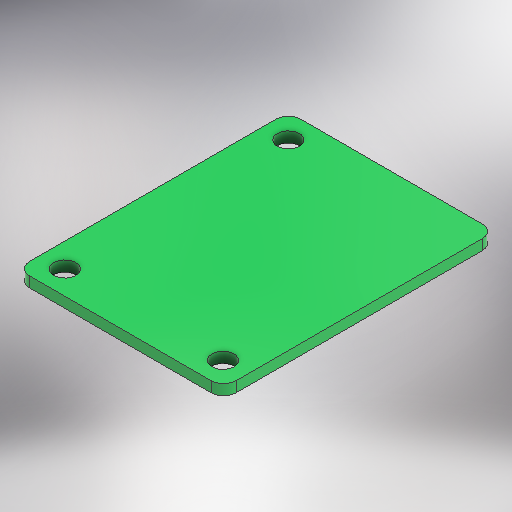
# Autodesk Inventor part: microphone_mcu
Saved by Autodesk Inventor 2026 (Build 300175050, 175E)
## iProperties
Created: 2025-06-24
Part Number: microphone_mcu
Material: Generic
Document SubType Name: Modeling
Designer: satom
Density: 1 g/cm^3
Appearance: Default
Author: satom
Autodesk Inventor part; units mm, degrees
ref_plane "YZ Plane" through (0, 0, 0) normal (1, 0, 0) x (0, 1, 0)
ref_plane "XZ Plane" through (0, 0, 0) normal (0, 1, 0) x (-1, 0, 0)
ref_plane "XY Plane" through (0, 0, 0) normal (0, 0, 1) x (1, 0, 0)
sketch "Sketch1" plane through (0, 0, 0) normal (0, 1, 0) x (-1, 0, 0)
  line L0 (13.895, 20.75) -> (-13.895, 20.75)
  line L1 (-15.8, 18.845) -> (-15.8, -18.845)
  line L2 (-13.895, -20.75) -> (13.895, -20.75)
  line L3 (15.8, -18.845) -> (15.8, 18.845)
  line L4 (15.8, 20.75) -> (-15.8, -20.75) construction
  line L5 (-15.8, 20.75) -> (15.8, -20.75) construction
  arc A0 (15.8, 18.845) -> (13.895, 20.75) centre (13.895, 18.845) ccw
  arc A1 (13.895, -20.75) -> (15.8, -18.845) centre (13.895, -18.845) ccw
  arc A2 (-15.8, -18.845) -> (-13.895, -20.75) centre (-13.895, -18.845) ccw
  arc A3 (-13.895, 20.75) -> (-15.8, 18.845) centre (-13.895, 18.845) ccw
  circle A4 centre (12.1, 17.15) radius 1.7
  circle A5 centre (12.1, -17.05) radius 1.7
  circle A6 centre (-12.1, 17.15) radius 1.7
  line L6 (15.8, 0) -> (-15.8, 0) construction
  point P0 (0, 0)
  dimension "d0" = 41.5
  dimension "d1" = 31.6
  dimension "d2" = 1.905
  dimension "d3" = 3.4
  dimension "d4" = 3.4
  dimension "d5" = 3.4
  dimension "d6" = 34.2
  dimension "d9" = 3.7
  dimension "d10" = 3.6
  dimension "d11" = 3.6
  dimension "d12" = 24.2
  dimension "d13" = 3.7
  constraints: 14 end point, 8 point on circle, 8 point on line, 8 tangent, 7 centre point, 4 midpoint, 3 equal radius, 2 parallel, 1 horizontal, 1 perpendicular
  measures "d0" distance of L5.start L4.end
  measures "d1" distance of L4.end L5.end
  measures "d2" radius of A0
  measures "d3" diameter of A4
  measures "d4" diameter of A5
  measures "d5" diameter of A6
  measures "d6" distance of A5.centre A4.centre
  measures "d9" distance from line of L2 A5.centre
  measures "d10" distance from line of L0 A4.centre
  measures "d11" distance from line of L0 A6.centre
  measures "d12" distance of A6.centre A4.centre
  measures "d13" distance from line of L3 A4.centre
extrude "Extrusion1" add sketch "Sketch1" along normal blind 1.6
equation "\"d3\" = m3_clearance"
equation "\"d4\" = d3"
equation "\"d5\" = d3"
equation "\"d11\" = d10"
equation "\"m3_heat_set_insert\" = 4"
equation "\"m3_clearance\" = 3.4"
equation "\"m3_heat_set_depth\" = 7"
equation "\"robot_diameter\" = 354"
equation "\"hardboard_thickness\" = 5"
equation "\"motor_centerline_height\" = 13"
body "Solid1"
